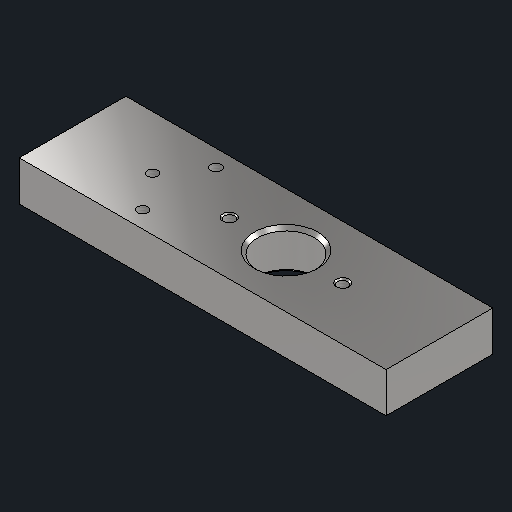
# Autodesk Inventor part: KN-00-02-11
Saved by Autodesk Inventor 2025.2 (Build 292293000, 293)
## iProperties
Created: 2025-04-25
Part Number: KN-00-02-11
Material: X5CrNi18-10
Document SubType Name: Modeling
Designer: Kacper Mik
Density: 8 g/cm^3
Appearance: Semi-Polished
Mass: 39.087 g
Surface Area: 27.4436 cm^2
Volume: 4.88588 cm^3
Author: Kacper Mik
Autodesk Inventor part; units mm, degrees
ref_plane "YZ Plane" through (0, 0, 0) normal (1, 0, 0) x (0, 1, 0)
ref_plane "XZ Plane" through (0, 0, 0) normal (0, 1, 0) x (-1, 0, 0)
ref_plane "XY Plane" through (0, 0, 0) normal (0, 0, 1) x (1, 0, 0)
sketch "Sketch1" plane through (0, 0, 0) normal (0, 1, 0) x (-1, 0, 0)
  line L0 (-27.5, 8) -> (27.5, 8)
  line L1 (27.5, 8) -> (27.5, -8)
  line L2 (27.5, -8) -> (-27.5, -8)
  line L3 (-27.5, -8) -> (-27.5, 8)
  line L4 (-27.5, 8) -> (27.5, -8) construction
  line L5 (27.5, 8) -> (-27.5, -8) construction
  point P0 (0, 0)
  dimension "d0" = 55
  dimension "d1" = 16
  constraints: 12 end point, 2 midpoint, 2 parallel, 1 horizontal, 1 perpendicular
  measures "d0" distance of L1.end L2.end
  measures "d1" distance of L2.end L0.start
extrude "Extrusion1" add sketch "Sketch1" along normal blind 6
sketch "Sketch2" plane through (0, 6, 0) normal (0, 1, 0) x (1, 0, 0)
  line L0 (27.5, 8) -> (-27.5, 8) construction
  line L1 (-27.5, 8) -> (-27.5, -8) construction
  line L2 (-27.5, -8) -> (27.5, -8) construction
  line L3 (27.5, -8) -> (27.5, 8) construction
  point P0 (0, 0)
  point P1 (4.5, 0)
  dimension "d4" = 23
  constraints: 1 horizontal alignment
  measures "d4" distance from line of L3 point (4.5, 0)
hole "Hole1" at (4.5, 6, 0) direction (0, -1, 0) diameter 8.5 end through all
chamfer "Chamfer1" distance 0.5 angle 45 2 edges at (4.5, 0, -4.25) (4.5, 6, -4.25)
sketch "Sketch3" plane through (0, 6, 0) normal (0, 1, 0) x (1, 0, 0)
  circle A0 centre (-15.5, 0) radius 1.4 construction
  line L0 (-18.5, 8) -> (-4.5, 8) construction
  line L1 (-4.5, 8) -> (-4.5, -8) construction
  line L2 (-4.5, -8) -> (-18.5, -8) construction
  line L3 (-18.5, 8) -> (-18.5, -8) projected
  circle A1 centre (-11.5, 5.5) radius 1.4 projected
  circle A2 centre (-11.5, -5.5) radius 1.4 projected
  point P0 (0, 0)
  point P1 (-15.5, 0)
  constraints: 3 coincident
hole "Hole2" at (-15.5, 6, 0) at (-11.5, 6, -5.5) at (-11.5, 6, 5.5) direction (0, -1, 0) diameter 1.567 end through all thread size "M2x0.4" class "6H" standard "ISO Metric profile"
chamfer "Chamfer2" distance 0.2 angle 45 3 edges at (-11.5, 0, -6.2835) (-15.5, 0, -0.7835) (-11.5, 0, 4.7165)
sketch "Sketch4" plane through (0, 6, 0) normal (0, 1, 0) x (1, 0, 0)
  circle A0 centre (-4, 0) radius 2.2 construction
  circle A1 centre (13, 0) radius 2.2 construction
  point P0 (0, 0)
  constraints: 2 coincident
hole "Hole3" at (-4, 6, 0) at (13, 6, 0) direction (0, -1, 0) diameter 1.567 end through all thread size "M2x0.4" class "6H" standard "ISO Metric profile"
chamfer "Chamfer3" distance 0.2 angle 45 2 edges at (13, 6, -0.7835) (-4, 6, -0.7835)
body "Solid1"
